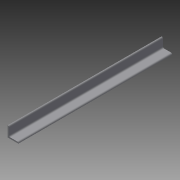
# Autodesk Inventor part: 2x2 quarter in angle aluminum
Saved by Autodesk Inventor 2015 (Build 190159000, 159)
## iProperties
Created: 2015-02-01
Part Number: 2x2 quarter in angle aluminum
Material: Generic
Document SubType Name: Modeling
Designer: szymsea16
Density: 1 g/cm^3
Appearance: Default
Author: szymsea16
Autodesk Inventor part; units mm, degrees
ref_plane "YZ Plane" through (0, 0, 0) normal (1, 0, 0) x (0, 1, 0)
ref_plane "XZ Plane" through (0, 0, 0) normal (0, 1, 0) x (-1, 0, 0)
ref_plane "XY Plane" through (0, 0, 0) normal (0, 0, 1) x (1, 0, 0)
sketch "Sketch1" plane through (0, 0, 0) normal (0, 1, 0) x (-1, 0, 0)
  line L0 (0, 0) -> (50.8, 0)
  line L1 (50.8, 0) -> (50.8, -736.6)
  line L2 (50.8, -736.6) -> (0, -736.6)
  line L3 (0, -736.6) -> (0, 0)
  dimension "d0" = 50.8
  dimension "d1" = 736.6
  constraints: 8 end point, 2 horizontal, 1 parallel, 1 perpendicular
  measures "d0" distance of L0.start L0.end
  measures "d1" distance of L0.end L1.end
extrude "Extrusion1" add sketch "Sketch1" along normal blind 6.35
sketch "Sketch2" plane through (0, 6.35, 0) normal (0, 1, 0) x (1, 0, 0)
  line L0 (-50.8, 0) -> (-44.45, 0)
  line L1 (-50.8, 0) -> (0, 0) projected
  line L2 (-44.45, 0) -> (-44.45, 736.6)
  line L3 (0, 736.6) -> (-50.8, 736.6) projected
  line L4 (-44.45, 736.6) -> (-50.8, 736.6)
  line L5 (-50.8, 736.6) -> (-50.8, 0)
  line L6 (-50.8, 0) -> (-44.45, 0)
  dimension "d4" = 6.35
  dimension "d5" = 736.6
  dimension "d6" = 736.6
  constraints: 10 end point, 1 perpendicular, 1 point on line, 1 vertical
  measures "d4" distance of L0.start L0.end
  measures "d5" distance of L0.end L2.end
  measures "d6" distance of L3.end L0.start
extrude "Extrusion2" add sketch "Sketch2" along normal blind 44.45
fillet "Fillet1" radius 6.35 1 edges at (-44.45, 6.35, -368.3)
fillet "Fillet2" radius 6.35 1 edges at (0, 6.35, -368.3)
fillet "Fillet3" radius 6.35 1 edges at (-44.45, 50.8, -368.3)
body "Solid1"
